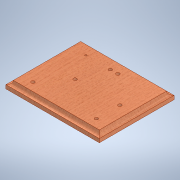
# Autodesk Inventor part: Wooden Base
Saved by Autodesk Inventor 2021.1 (Build 251245010, 245A)
## iProperties
Created: 2025-09-16
Material: Wood (Oak)
Document SubType Name: Modeling
Designer: SD
Density: 0.76 g/cm^3
Appearance: White Oak - Natural Medium Gloss
Mass: 695.072 g
Surface Area: 1183.36 cm^2
Volume: 914.569 cm^3
Project: Automatic Tea Steeping mechanism
Part Number: Wooden Base
Length: 200.000 mm
Thickness: 20.000 mm
Width: 250.000 mm
BOM-Mass: 0.69507
BOM-Area: 0.118
Author: SD
Title: Wooden Base
Autodesk Inventor part; units mm, degrees
ref_plane "YZ Plane" through (0, 0, 0) normal (1, 0, 0) x (0, 1, 0)
ref_plane "XZ Plane" through (0, 0, 0) normal (0, 1, 0) x (-1, 0, 0)
ref_plane "XY Plane" through (0, 0, 0) normal (0, 0, 1) x (1, 0, 0)
sketch "Sketch1" plane through (0, 0, 0) normal (0, 0, 1) x (1, 0, 0)
  line L0 (-125, 10) -> (125, 10)
  line L1 (125, 10) -> (125, -10)
  line L2 (125, -10) -> (-125, -10)
  line L3 (-125, -10) -> (-125, 10)
  line L4 (-125, 10) -> (125, -10) construction
  line L5 (125, 10) -> (-125, -10) construction
  point P0 (0, 0)
  constraints: 12 end point, 4 parallel, 2 midpoint, 1 horizontal, 1 perpendicular
extrude "Extrusion1" add sketch "Sketch1" along normal mid plane 200
fillet "Fillet1" radius 10 4 edges at (125, 10, 0) (0, 10, 100) (-125, 10, 0) (0, 10, -100) inverted yes
sketch "Sketch2" plane through (-115, 10, -90) normal (0, 1, 0) x (1, 0, 0)
  line L0 (-10, 10) -> (-10, -190) projected
  line L1 (240, 10) -> (-10, 10) projected
  line L2 (240, -190) -> (240, 10) projected
  point P0 (115, -90)
  point P1 (105, -25.5)
  point P2 (125, -25.5)
  point P3 (80, -95)
  point P4 (200, -95)
  point P5 (30, -158)
  point P6 (200, -158)
  dimension "d5" = 115
  dimension "d6" = 20
  dimension "d7" = 35.5
  dimension "d8" = 105
  dimension "d9" = 40
  dimension "d10" = 120
  dimension "d11" = 168
  dimension "d12" = 40
  dimension "d13" = 170
  constraints: 3 horizontal alignment
  measures "d5" distance from line of point (105, -25.5) L0
  measures "d6" distance of point (125, -25.5) point (105, -25.5)
  measures "d7" distance from line of point (105, -25.5) L1
  measures "d8" distance from line of point (200, -95) L1
  measures "d9" distance from line of L2 point (200, -95)
  measures "d10" distance of point (80, -95) point (200, -95)
  measures "d11" distance from line of point (200, -158) L1
  measures "d12" distance from line of L2 point (200, -158)
  measures "d13" distance of point (200, -158) point (30, -158)
hole "Hole1" at (-10, 10, -64.5) at (10, 10, -64.5) at (-35, 10, 5) at (85, 10, 5) at (-85, 10, 68) at (85, 10, 68) direction (0, -1, 0) diameter 9 depth 20
sketch "Sketch3" plane through (-125, -10, 100) normal (0, -1, 0) x (1, 0, 0)
  circle A0 centre (40, -32) radius 4.5 projected
  circle A1 centre (90, -95) radius 4.5 projected
  circle A2 centre (210, -32) radius 4.5 projected
  circle A3 centre (210, -95) radius 4.5 projected
  circle A4 centre (135, -164.5) radius 4.5 projected
  circle A5 centre (115, -164.5) radius 4.5 projected
  point P0 (125, -100)
  constraints: 6 coincident
hole "Hole2" at (-85, -10, 68) at (-35, -10, 5) at (85, -10, 68) at (85, -10, 5) at (10, -10, -64.5) at (-10, -10, -64.5) direction (0, 1, 0) diameter 16.1 depth 10.1
sketch "Sketch4" plane through (-115, 10, -90) normal (0, 1, 0) x (1, 0, 0)
  line L0 (-10, 10) -> (-10, -190) projected
  line L1 (240, 10) -> (-10, 10) projected
  point P0 (115, -90)
  point P1 (39, -25)
  dimension "d28" = 49
  dimension "d30" = 35
  measures "d28" distance from line of point (39, -25) L0
  measures "d30" distance from line of L1 point (39, -25)
hole "Hole3" at (-76, 10, -65) direction (0, -1, 0) diameter 5 depth 20 tip angle 118
sketch "Sketch7" plane through (-125, -10, 100) normal (0, -1, 0) x (1, 0, 0)
  circle A0 centre (49, -165) radius 2.5 projected
  point P0 (125, -100)
  constraints: 1 coincident
hole "Hole5" at (-76, -10, -65) direction (0, 1, 0) diameter 9.1 depth 5.3
body "Solid1"
